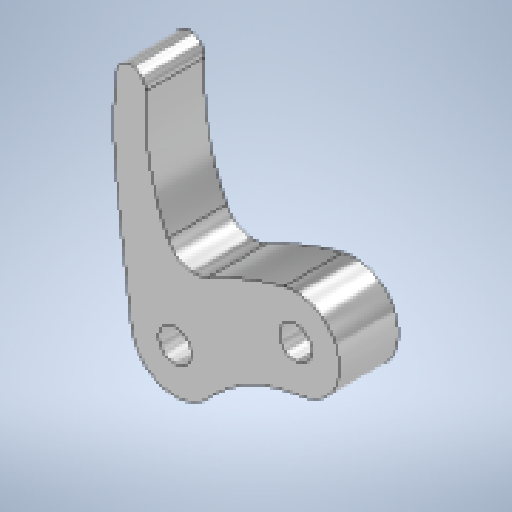
# Autodesk Inventor part: Lever
Saved by Autodesk Inventor 2023.2 (Build 272271000, 271)
## iProperties
Created: 2024-01-16
Part Number: Lever
Material: Aluminum 6061
Document SubType Name: Modeling
Designer: Nathan Cai
Mass: 4.74857 g
Surface Area: 12.8388 cm^2
Volume: 1.75873 cm^3
Density: 2.7 g/cm^3
Appearance: Aluminum - Flat
Author: Nathan Cai
Autodesk Inventor part; units mm, degrees
ref_plane "YZ Plane" through (0, 0, 0) normal (1, 0, 0) x (0, 1, 0)
ref_plane "XZ Plane" through (0, 0, 0) normal (0, 1, 0) x (-1, 0, 0)
ref_plane "XY Plane" through (0, 0, 0) normal (0, 0, 1) x (1, 0, 0)
sketch "Sketch1" plane through (0, 0, 0) normal (0, 0, 1) x (1, 0, 0)
  circle A0 centre (0, 0) radius 1.7526
  circle A1 centre (0, 0) radius 4.7625
  circle A2 centre (0, 0) radius 19.05 construction
  circle A3 centre (0, 19.05) radius 3.175 construction
  line L0 (0, 19.05) -> (0, 0) construction
  line L1 (0, 19.05) -> (3.175, 19.05) construction
  arc A4 (-3.1628, 22.1199) -> (-6.3202, 22.4358) centre (-4.7468, 22.225) ccw
  arc A5 (-6.3202, 22.4358) -> (-6.3695, 12.7) centre (31.4424, 17.3766) ccw
  line L2 (-6.3695, 12.7) -> (-4.7265, -0.5846)
  circle A6 centre (12.9789, 6.7647) radius 6.35 construction
  line L3 (6.8453, 5.1212) -> (12.9789, 6.7647) construction
  line L4 (0, 0) -> (-2.3924, 8.9287) construction
  circle A7 centre (12.9789, 6.7647) radius 1.7526
  circle A8 centre (12.9789, 6.7647) radius 4.7625
  arc A9 (-3.1628, 22.1199) -> (3.5023, 3.2272) centre (22.1815, 20.4391) ccw
  arc A10 (11.7463, 11.3649) -> (-3.0649, 3.6452) centre (21.71, -25.8202) ccw
  line L5 (11.7463, 11.3649) -> (7.6893, 10.2778) construction
  arc A11 (13.5395, 2.0353) -> (3.5557, -3.1683) centre (15.4082, -13.7293) ccw
  circle A12 centre (4.7625, -9.525) radius 6.35 construction
  circle A13 centre (4.7625, -9.525) radius 1.7526
  circle A14 centre (4.7625, -9.525) radius 4.7625
  arc A15 (13.6466, 2.0492) -> (8.9515, -7.2592) centre (14.5368, -4.2381) ccw
  arc A16 (-4.7466, -0.3889) -> (1.6034, -13.0889) centre (14.2398, 1.1668) ccw
  arc A17 (8.516, 5.1021) -> (3.4469, -4.9478) centre (14.5368, -4.2381) ccw
  arc A18 (1.1746, -4.6154) -> (1.7749, -5.8161) centre (14.2398, 1.1668) ccw
  arc A19 (8.4772, 5.2104) -> (3.8525, 2.8) centre (21.71, -25.8202) ccw
  circle A20 centre (0, 0) radius 3.175 construction
  point P0 (3.7177, 2.9766)
  point P1 (0.9028, 6.5691)
  point P2 (3.4669, -3.2653)
  point P3 (-4.7377, -0.494)
  dimension "d1" = 9.525
  dimension "d2" = 38.1
  dimension "d3" = 6.35
  dimension "d0" = 3.5052
  dimension "d5" = 3.175
  dimension "d6" = 3.175
  dimension "d7" = 38.1
  dimension "d8" = 6.35
  dimension "d11" = 12.7
  dimension "d12" = 3.5052
  dimension "d13" = 14.2875
  dimension "d14" = 3.175
  dimension "d16" = 9.525
  dimension "d18" = 25.4
  dimension "d19" = 15.875
  dimension "d21" = 12.7
  dimension "d22" = 3.5052
  dimension "d23" = 9.525
  dimension "d24" = 4.7625
  dimension "d25" = 9.525
  dimension "d26" = 6.35
  dimension "d27" = 4.7625
  dimension "d28" = 4.7625
  dimension "d29" = 4.7625
  dimension "d31" = 19.05
  dimension "d32" = 15
  dimension "d33" = 6.35
  constraints: 32 point on circle, 18 centre point, 12 end point, 10 tangent, 8 coincident, 1 horizontal, 1 horizontal alignment, 1 parallel, 1 perpendicular, 1 vertical, 1 vertical alignment, 20 other
  measures "d0" diameter of A0
  measures "d5" diameter of A4
  measures "d6" distance from line of L1 A4.centre
  measures "d7" radius of A5
  measures "d8" distance from line of L1 L2.start
  measures "d11" diameter of A6
  measures "d12" diameter of A7
  measures "d13" distance from line of L4 L3.end
  measures "d14" distance from line of point (0, 0) L3
  measures "d16" diameter of A8
  measures "d18" radius of A9
  measures "d19" radius of A11
  measures "d21" diameter of A12
  measures "d22" diameter of A13
  measures "d23" vertical distance of A13.centre point (0, 0)
  measures "d24" horizontal distance of A0.centre A13.centre
  measures "d25" diameter of A14
  measures "d26" radius of A15
  measures "d27" radial gap between concentric circles of A15 A17
  measures "d28" radial gap between concentric circles of A16 A18
  measures "d29" radial gap between concentric circles of A10 A19
  measures "d31" radius of A16
  measures "d32" angle of L0 L4
  measures "d33" diameter of A20
extrude "Extrusion1" add sketch "Sketch1" along normal blind 6.35 contours A1 A17 | A19 A8 A17 A1 | A1 A9 A10 A8 A19 | A1 A10 A9 | A17 A8 A11 A1 | A1 A17 | A8 | A1 L2 A5 A4 A9 A10
fillet "Fillet1" radius 3.175 1 edges at (0.9028, 6.5691, 3.175)
fillet "Fillet2" [suppressed]
fillet "Fillet3" [suppressed]
body "Solid1"
